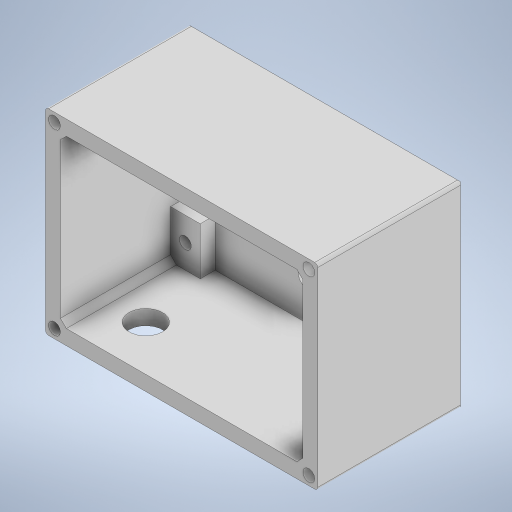
# Autodesk Inventor part: boitierPCB
Saved by Autodesk Inventor 2024 (Build 280153000, 153)
## iProperties
Created: 2023-07-12
Part Number: boitierPCB
Material: Generic
Document SubType Name: Modeling
Designer: pablo
Density: 1 g/cm^3
Appearance: Default
Author: pablo
Autodesk Inventor part; units mm, degrees
ref_plane "YZ Plane" through (0, 0, 0) normal (1, 0, 0) x (0, 1, 0)
ref_plane "XZ Plane" through (0, 0, 0) normal (0, 1, 0) x (-1, 0, 0)
ref_plane "XY Plane" through (0, 0, 0) normal (0, 0, 1) x (1, 0, 0)
sketch "Sketch1" plane through (0, 0, 0) normal (0, 0, 1) x (1, 0, 0)
  line L0 (0, 0) -> (-91.5, 0)
  line L1 (-91.5, 0) -> (-91.5, 66)
  line L2 (-91.5, 66) -> (0, 66)
  line L3 (0, 66) -> (0, 0)
  point P0 (-45.75, 66)
  dimension "d1" = 66
  dimension "d2" = 91.5
  constraints: 8 end point, 2 parallel, 1 horizontal, 1 midpoint, 1 perpendicular
  measures "d1" distance from line of point (-45.75, 66) L0
  measures "d2" distance of L0.start L0.end
extrude "Extrusion1" add sketch "Sketch1" along normal blind 50
sketch "Sketch2" plane through (0, 0, 50) normal (0, 0, 1) x (1, 0, 0)
  line L0 (-86.5, 61) -> (-5, 61)
  line L1 (-5, 61) -> (-5, 5)
  line L2 (-5, 5) -> (-86.5, 5)
  line L3 (-86.5, 5) -> (-86.5, 61)
  line L4 (0, 66) -> (-91.5, 66) projected
  line L5 (0, 0) -> (0, 66) projected
  line L6 (-91.5, 0) -> (0, 0) projected
  line L7 (-91.5, 66) -> (-91.5, 0) projected
  dimension "d5" = 5
  dimension "d6" = 5
  dimension "d7" = 5
  dimension "d8" = 5
  constraints: 8 end point, 2 parallel, 1 horizontal, 1 perpendicular
  measures "d5" distance between parallel lines of L4 L0
  measures "d6" distance between parallel lines of L5 L1
  measures "d7" distance between parallel lines of L6 L2
  measures "d8" distance between parallel lines of L7 L3
extrude "Extrusion2" cut sketch "Sketch2" against normal blind 42 contours L0 L1 L2 L3
sketch "Sketch3" plane through (0, 0, 8) normal (0, 0, 1) x (1, 0, 0)
  line L0 (-5, 5) -> (-86.5, 5) projected
  line L1 (-86.5, 61) -> (-5, 61) projected
  line L2 (-86.5, 5) -> (-5, 61)
  line L3 (-5, 5) -> (-86.5, 61)
  line L4 (-45.75, 48) -> (-60.75, 33)
  line L5 (-60.75, 33) -> (-45.75, 18)
  line L6 (-45.75, 18) -> (-30.75, 33)
  line L7 (-45.75, 48) -> (-45.75, 18)
  line L8 (-30.75, 33) -> (-60.75, 33)
  line L9 (-45.75, 48) -> (-30.75, 33)
  line L10 (-45.75, 33) -> (-45.75, 61)
  point P0 (0, 0)
  dimension "d11" = 30
  constraints: 18 end point, 4 coincident, 4 perpendicular, 3 midpoint, 1 collinear
  measures "d11" distance of L4.start L5.end
hole "Hole1" at (-45.75, 48, 8) at (-60.75, 33, 8) at (-45.75, 18, 8) at (-30.75, 33, 8) direction (0, 0, -1) diameter 5.6 end through all
sketch "Sketch5" plane through (0, 0, 8) normal (0, 0, 1) x (1, 0, 0)
  line L0 (-55.91, 43.16) -> (-35.59, 43.16)
  line L1 (-35.59, 43.16) -> (-35.59, 22.84)
  line L2 (-35.59, 22.84) -> (-55.91, 22.84)
  line L3 (-55.91, 22.84) -> (-55.91, 43.16)
  line L4 (-35.59, 43.16) -> (-55.91, 22.84)
  line L5 (-55.91, 43.16) -> (-35.59, 22.84)
  line L6 (-86.5, 61) -> (-5, 61) projected
  line L7 (-5, 5) -> (-86.5, 5) projected
  line L8 (-86.5, 61) -> (-5, 5)
  line L9 (-5, 61) -> (-86.5, 5)
  point P0 (0, 0)
  point P1 (-45.75, 33)
  dimension "d26" = 20.32
  dimension "d27" = 20.32
  constraints: 16 end point, 4 coincident, 2 midpoint, 2 parallel, 1 horizontal, 1 perpendicular
  measures "d26" distance between parallel lines of L2 L0
  measures "d27" distance between parallel lines of L1 L3
hole "Hole3" at (-55.91, 43.16, 8) at (-35.59, 43.16, 8) at (-35.59, 22.84, 8) at (-55.91, 22.84, 8) direction (0, 0, -1) diameter 4 depth 8 tip angle 118
sketch "Sketch6" plane through (0, 0, 50) normal (0, 0, 1) x (1, 0, 0)
  line L0 (-5, 5) -> (-86.5, 5) projected
  line L1 (-86.5, 5) -> (-85.5, 5)
  line L2 (-85.5, 5) -> (-85.5, 6)
  line L3 (-85.5, 6) -> (-86.5, 6)
  line L4 (-86.5, 6) -> (-86.5, 5)
  line L5 (-5, 61) -> (-5, 5) projected
  line L6 (-5, 6) -> (-6, 6)
  line L7 (-6, 6) -> (-6, 5)
  line L8 (-6, 5) -> (-5, 5)
  line L9 (-5, 5) -> (-5, 6)
  line L10 (-5, 60) -> (-6, 60)
  line L11 (-6, 60) -> (-6, 61)
  line L12 (-6, 61) -> (-5, 61)
  line L13 (-5, 61) -> (-5, 60)
  line L14 (-85.5, 61) -> (-86.5, 61)
  line L15 (-86.5, 61) -> (-86.5, 60)
  line L16 (-86.5, 60) -> (-85.5, 60)
  line L17 (-85.5, 60) -> (-85.5, 61)
  point P0 (0, 0)
  point P1 (-85.5, 5.5)
  dimension "d35" = 1
  dimension "d36" = 1
  dimension "d37" = 1
  dimension "d38" = 1
  dimension "d39" = 1
  dimension "d40" = 1
  dimension "d41" = 1
  constraints: 32 end point, 8 parallel, 7 point on line, 4 horizontal, 4 perpendicular, 1 midpoint
  measures "d35" distance from line of L4 point (-85.5, 5.5)
  measures "d36" distance between parallel lines of L0 L3
  measures "d37" distance between parallel lines of L14 L16
  measures "d38" distance between parallel lines of L15 L17
  measures "d39" distance between parallel lines of L13 L11
  measures "d40" distance between parallel lines of L12 L10
  measures "d41" distance between parallel lines of L0 L6
extrude "Extrusion3" add sketch "Sketch6" against normal through all
sketch "Sketch7" plane through (0, 0, 50) normal (0, 0, 1) x (1, 0, 0)
  line L0 (-85.5, 60) -> (-86.5, 60) projected
  line L1 (-91.5, 66) -> (-91.5, 0) projected
  line L2 (-85.5, 60) -> (-91.5, 66)
  line L3 (-85.5, 5) -> (-85.5, 6) projected
  line L4 (-85.5, 6) -> (-91.5, 0)
  line L5 (0, 0) -> (-6, 6)
  line L6 (0, 66) -> (-91.5, 66) projected
  line L7 (-6, 60) -> (-6, 61) projected
  line L8 (0, 66) -> (-6, 60)
  line L9 (0, 0) -> (0, 66) projected
  line L10 (-91.5, 0) -> (0, 0) projected
  point P0 (-3, 63)
  point P1 (-88.5, 63)
  point P2 (-88.5, 3)
  point P3 (-3, 3)
  point P4 (-3, 3)
  dimension "d44" = 3
  dimension "d45" = 3
  constraints: 8 end point, 5 midpoint, 1 perpendicular
  measures "d44" distance from line of L9 point (-3, 3)
  measures "d45" distance from line of L10 point (-3, 3)
hole "Hole4" at (-3, 63, 50) at (-88.5, 63, 50) at (-88.5, 3, 50) at (-3, 3, 50) direction (0, 0, -1) diameter 4 depth 10 tip angle 118
sketch "Sketch8" plane through (-91.5, 0, 0) normal (0, -1, 0) x (1, 0, 0)
  line L0 (91.5, 0) -> (91.5, 50) projected
  line L1 (0, 0) -> (91.5, 0) projected
  point P0 (18.5, 34.8)
  point P1 (91.5, 25)
  dimension "d75" = 73
  dimension "d76" = 34.8
  constraints: 1 midpoint
  measures "d75" horizontal distance of point (91.5, 25) point (18.5, 34.8)
  measures "d76" distance from line of L1 point (18.5, 34.8)
hole "Hole5" at (-73, 0, 34.8) direction (0, 1, 0) diameter 11.3 depth 10 tip angle 118
sketch "Sketch10" plane through (0, 0, 8) normal (0, 0, 1) x (1, 0, 0)
  line L0 (-6, 5) -> (-85.5, 5) projected
  line L1 (-86.5, 6) -> (-86.5, 60) projected
  line L2 (-76.5, 5) -> (-86.5, 5)
  line L3 (-86.5, 5) -> (-86.5, 33)
  line L4 (-86.5, 21) -> (-76.5, 21)
  line L5 (-76.5, 21) -> (-76.5, 5)
  line L6 (-5, 60) -> (-5, 6) projected
  line L7 (-15, 5) -> (-5, 5)
  line L8 (-5, 5) -> (-5, 33)
  line L9 (-5, 21) -> (-15, 21)
  line L10 (-15, 21) -> (-15, 5)
  point P0 (0, 0)
  point P1 (-5, 21)
  dimension "d71" = 10
  dimension "d72" = 10
  dimension "d85" = 16
  dimension "d86" = 16
  constraints: 16 end point, 4 parallel, 2 horizontal, 2 midpoint, 2 perpendicular, 2 point on line
  measures "d71" distance between parallel lines of L1 L5
  measures "d72" distance between parallel lines of L6 L10
  measures "d85" distance between parallel lines of L0 L9
  measures "d86" distance between parallel lines of L0 L4
extrude "Extrusion4" add sketch "Sketch10" along normal blind 5
sketch "Sketch9" plane through (0, 0, 8) normal (0, 0, 1) x (1, 0, 0)
  line L0 (-6, 5) -> (-85.5, 5) projected
  line L1 (-86.5, 6) -> (-86.5, 60) projected
  point P0 (0, 0)
  point P1 (-10, 13)
  point P2 (-81.5, 13)
  dimension "d67" = 8
  dimension "d68" = 8
  dimension "d69" = 71.5
  dimension "d70" = 5
  measures "d67" distance from line of L0 point (-81.5, 13)
  measures "d68" distance from line of L0 point (-10, 13)
  measures "d69" distance of point (-81.5, 13) point (-10, 13)
  measures "d70" distance from line of L1 point (-81.5, 13)
hole "Hole6" at (-10, 13, 8) at (-81.5, 13, 8) direction (0, 0, -1) diameter 4 end through all both
chamfer "Chamfer1" distance 2 angle 45 4 edges at (-45.75, 0, 0) (-91.5, 33, 0) (-45.75, 66, 0) (0, 33, 0)
fillet "Fillet2" radius 1 4 edges at (0, 0, 26) (-91.5, 0, 26) (-91.5, 66, 26) (0, 66, 26)
chamfer "Chamfer2" distance 1 angle 45 8 edges at (-86.5, 6, 31.5) (-85.5, 5, 31.5) (-86.5, 60, 29) (-85.5, 61, 29) (-6, 5, 31.5) (-5, 6, 31.5) (-6, 61, 29) (-5, 60, 29)
body "Solid1"
